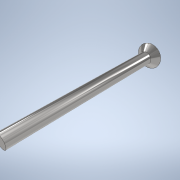
# Autodesk Inventor part: Армирующий сопло гвоздик
Saved by Autodesk Inventor 2021.1 (Build 251245010, 245A)
## iProperties
Created: 2026-05-28
Part Number: Армирующий сопло гвоздик
Material: Типовые
Document SubType Name: Modeling
Designer: Андрей Тарасов
Density: 1 g/cm^3
Appearance: По умолчанию
Author: Андрей Тарасов
Autodesk Inventor part; units mm, degrees
ref_plane "YZ Plane" through (0, 0, 0) normal (1, 0, 0) x (0, 1, 0)
ref_plane "XZ Plane" through (0, 0, 0) normal (0, 1, 0) x (-1, 0, 0)
ref_plane "XY Plane" through (0, 0, 0) normal (0, 0, 1) x (1, 0, 0)
sketch "Эскиз1" plane through (0, 0, 0) normal (1, 0, 0) x (0, 1, 0)
  line L0 (0, 0) -> (1, 0)
  line L1 (1, 0) -> (1, -24)
  line L2 (1, -24) -> (2, -25)
  line L3 (2, -25) -> (0, -25)
  line L4 (0, -25) -> (0, 0)
  dimension "d1" = 1
  dimension "d2" = 25
  dimension "d3" = 24
  dimension "d4" = 2
  constraints: 10 end point, 2 horizontal, 1 parallel, 1 vertical
  measures "d1" distance between parallel lines of L4 L1
  measures "d2" distance from line of L0.start L3
  measures "d3" distance of L0.end L1.end
  measures "d4" distance of L2.end L3.end
revolve "Вращение1" add sketch "Эскиз1" angle 360 about axis through (0, 0, -25) along (0, 0, 1)
